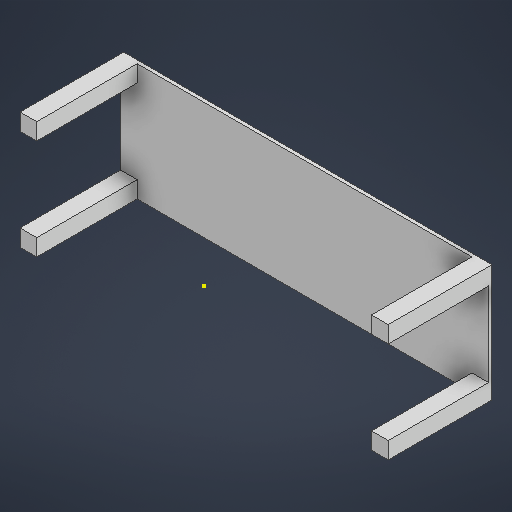
# Autodesk Inventor part: table
Saved by Autodesk Inventor 2027 (Build 310192060, 192F)
## iProperties
Created: 2026-07-29
Part Number: table
Material: 일반
Document SubType Name: Modeling
Designer: duqck
Density: 1 g/cm^3
Appearance: 기본값
Author: duqck
Autodesk Inventor part; units mm, degrees
ref_plane "YZ Plane" through (0, 0, 0) normal (1, 0, 0) x (0, 1, 0)
ref_plane "XZ Plane" through (0, 0, 0) normal (0, 1, 0) x (-1, 0, 0)
ref_plane "XY Plane" through (0, 0, 0) normal (0, 0, 1) x (1, 0, 0)
sketch "스케치1" plane through (0, 0, 0) normal (0, 0, 1) x (1, 0, 0)
  line L0 (-550, 175) -> (550, 175)
  line L1 (550, 175) -> (550, -175)
  line L2 (550, -175) -> (-550, -175)
  line L3 (-550, -175) -> (-550, 175)
  point P0 (0, 0)
  point P1 (550, 0)
  dimension "d0" = 1100
  dimension "d1" = 350
  dimension "d8" = 550
  dimension "d9" = 175
  constraints: 8 end point, 2 parallel, 1 horizontal, 1 midpoint, 1 perpendicular
  measures "d0" distance of L0.start L0.end
  measures "d1" distance of L2.end L0.start
  measures "d8" distance of point (550, 0) point (0, 0)
  measures "d9" distance from line of L2 point (0, 0)
extrude "돌출1" add sketch "스케치1" along normal mid plane 10
sketch "스케치2" plane through (0, 0, 5) normal (0, 0, 1) x (1, 0, 0)
  line L0 (550, -175) -> (550, 175) projected
  line L1 (550, -175) -> (500, -175)
  line L2 (500, -175) -> (500, -125)
  line L3 (500, -125) -> (550, -125)
  line L4 (550, -125) -> (550, -175)
  point P0 (0, 0)
  dimension "d4" = 50
  dimension "d5" = 50
  constraints: 8 end point, 2 parallel, 1 horizontal, 1 perpendicular
  measures "d4" distance of L2.end L3.end
  measures "d5" distance of L1.end L2.end
extrude "돌출2" add sketch "스케치2" along normal blind 300
sketch "스케치3" plane through (0, 0, 305) normal (0, 0, 1) x (1, 0, 0)
  point P0 (0, 0)
mirror "미러1" about plane through (0, 0, 0) normal (0, 1, 0) of "돌출2"
mirror "미러2" about plane through (0, 0, 0) normal (1, 0, 0) of "돌출2", "미러1"
equation "\"d8\" = 0.5 * d0"
equation "\"d9\" = 0.5 * d1"
